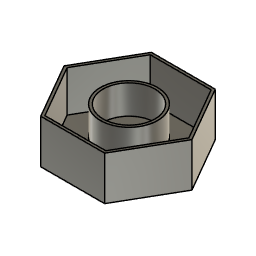
10403김동현_스케치 v1 (Autodesk Fusion 360 design; units mm, degrees)
Autodesk Fusion 360 part; units mm, degrees
note: some values were not read from the file. Chosen so that the rebuilt part matches the saved one: which bodies a step acts on.
sketch "스케치1" plane through (0, 0, 0) normal (0, 0, 1) x (1, 0, 0)
  line L0 (-99.9274, 68.1306) -> (-63.4299, 131.4121)
  line L1 (-63.4299, 131.4121) -> (-99.9846, 194.6607)
  line L2 (-99.9846, 194.6607) -> (-173.0368, 194.6277)
  line L3 (-173.0368, 194.6277) -> (-209.5343, 131.3462)
  line L4 (-209.5343, 131.3462) -> (-172.9796, 68.0976)
  line L5 (-172.9796, 68.0976) -> (-99.9274, 68.1306)
  point P0 (-136.4821, 131.3792)
extrude "돌출1" add sketch "스케치1" along normal blind 50 makes body 1
sketch "스케치2" plane through (0, 0, 50) normal (0, 0, 1) x (-1, 0, 0)
  circle A0 centre (134.6748, -130.7023) radius 29.6684
extrude "돌출2" cut sketch "스케치2" against normal blind 30 bodies 1
shell "쉘1" thickness 3 removed faces 1 at (-181.3254, 156.5162, 50) on bodies 1 makes body 2 at (-148.6479, 110.2853, 0)
delete_face "면 삭제1" 1 faces at (-141.7097, 117.2056, 20) on bodies 1
